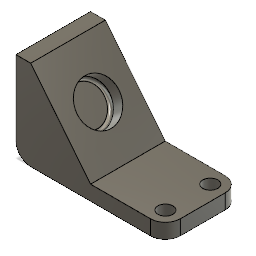
3.9 move and copy (Autodesk Fusion 360 design; units mm, degrees)
Autodesk Fusion 360 part; units mm, degrees
sketch "Sketch1" plane through (0, 0, 0) normal (0, 0, 1) x (1, 0, 0)
  line L0 (0, 6) -> (0, 1)
  line L1 (1, 0) -> (10, 0)
  line L2 (10, 0) -> (10, 1)
  line L3 (10, 1) -> (5, 1)
  line L4 (5, 1) -> (1, 6)
  line L5 (1, 6) -> (0, 6)
  arc A0 (0, 1) -> (1, 0) centre (1, 1) ccw
  dimension "d1" = 6
  dimension "d2" = 10
  dimension "d3" = 1
  dimension "d4" = 5
  dimension "d5" = 1
  dimension "d6" = 1
  measures "d1" distance of origin
  measures "d2" distance of origin
  measures "d3" radius of A0
extrude "Extrude1" add sketch "Sketch1" along normal blind 5
sketch "Sketch2" plane through (3.5366, 2.8293, 0) normal (0.780869, 0.624695, 0) x (0, 0, -1)
  line L0 (0, -2.3426) -> (0, 4.0605)
  line L1 (0, 4.0605) -> (-5, 4.0605)
  line L2 (-5, 4.0605) -> (-5, -2.3426)
  line L3 (-5, -2.3426) -> (0, -2.3426)
  circle A0 centre (-2.5, 0.8605) radius 1.4
  dimension "d9" = 2.8
  dimension "d10" = 3.2
  dimension "d11" = 2.5
  measures "d9" diameter of A0
  measures "d10" distance of L1
  measures "d11" distance of L0
extrude "Extrude2" cut sketch "Sketch2" against normal blind 1 contours A0
fillet "Fillet1" radius 0.2 1 edges at (1.9019, 3.2718, 3.8053)
fillet "Fillet2" radius 1 1 edges at (10, 0.5, 5)
fillet "Fillet3" radius 1 1 edges at (10, 0.5, 0)
sketch "Sketch3" plane through (0, 1, 0) normal (0, 1, 0) x (-1, 0, 0)
  arc A0 (-10, 1) -> (-9, 0) centre (-9, 1) ccw
  line L0 (-9, 0) -> (-5, 0)
  line L1 (-5, 0) -> (-5, 5)
  line L2 (-5, 5) -> (-9, 5)
  arc A1 (-9, 5) -> (-10, 4) centre (-9, 4) ccw
  line L3 (-10, 4) -> (-10, 1)
  circle A2 centre (-9, 1) radius 0.5
  circle A3 centre (-9, 4) radius 0.5
  dimension "d17" = 1
  dimension "d18" = 1
  dimension "d19" = 4
  measures "d17" diameter of A2
  measures "d18" diameter of A3
  measures "d19" distance of L1
extrude "Extrude3" cut sketch "Sketch3" against normal through all contours A2 | A3
